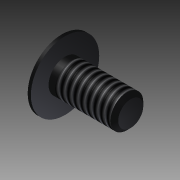
# Autodesk Inventor part: 3342
Saved by Autodesk Inventor 2016 (Build 200138000, 138)
## iProperties
Category: PARTsolutions
Company: 8020
Created: 2016-04-17
Part Number: 3342
Catalog Web Link: www.cadenas.de
Description: 3390, 3342, 3066, 3340, 3330-Flanged Button Head Socket Cap Screws
Vendor: 8020
Document SubType Name: Modeling
Designer: psAdmin
Manufacturer: 8020
Mass: 0.617423 g
Surface Area: 6.01161 cm^2
Volume: 0.617423 cm^3
Density: 1 g/cm^3
Material: Generic
Appearance: PSOLRGB-0-0-0
PSOL_IDENT_0: {$CADENAS_DATA\23d-libs\8020\inch\fastening_options\3390.prj},164 {VTYP=3D},{NB=3342},{LINA=3342},{N
PSOL_IDENT_1: N=3390, 3342, 3066, 3340, 3330},{DATE=22.08.2012},{GEOMDATE=11.05.2012 00:00:00},{VERSION=},{LINEID=
PSOL_IDENT_2: 10},{LINESUBID=-1},{WBVAR=L}  {NB=3342},{LINA=3342},{KT=DUMMY},{PN=3342},{FIN=Black Zinc},{THRD=1/4-
PSOL_IDENT_3: 20},{THRD1=0.2500},{L=0.50000000},{L1=0.375,0.5,0.75},{W=.009},{A=0.120},{D=0.520},{S=0.160},{T=0.09
PSOL_IDENT_4: 0}
NN: 3390, 3342, 3066, 3340, 3330
NT: Flanged Button Head Socket Cap Screws
NB: 3342
NBSYN: $PN.
LINA: 3342
PN: 3342
FIN: Black Zinc
THRD: 1/4-20
L: 1/2
W: .009
SUPPLIER: 8020
ARTICLENO: 3342
BOMINFO: 3342
CREATOR: CADENAS GmbH
Title: 3342
Author: Cadenas PARTsolutions
Comments: Flanged Button Head Socket Cap Screws
Autodesk Inventor part; units mm, degrees
ref_plane "YZ Plane" through (0, 0, 0) normal (1, 0, 0) x (0, 1, 0)
ref_plane "XZ Plane" through (0, 0, 0) normal (0, 1, 0) x (-1, 0, 0)
ref_plane "XY Plane" through (0, 0, 0) normal (0, 0, 1) x (1, 0, 0)
sketch "Sketch_1" plane through (0, 0, 0) normal (0, 0, 1) x (1, 0, 0)
  line L0 (12.7, 0) -> (-3.048, 0)
  line L1 (-3.048, 0) -> (-3.048, 2.4384)
  arc A0 (-0.6096, 5.9436) -> (-3.048, 2.4384) centre (3.3013, 0.6222) ccw
  line L2 (-0.6096, 5.9436) -> (-0.6096, 6.604)
  line L3 (-0.6096, 6.604) -> (0, 6.604)
  line L4 (0, 6.604) -> (0, 3.175)
  line L5 (0, 3.175) -> (11.9444, 3.175)
  line L6 (11.9444, 3.175) -> (12.7, 2.4194)
  line L7 (12.7, 2.4194) -> (12.7, 0)
  line L8 (12.7, 0) -> (-3.048, 0)
  constraints: 18 end point, 2 point on circle, 1 centre point
revolve "Revolution1" add sketch "Sketch_1" angle 360 about axis through (12.7, 0, 0) along (1, 0, 0)
thread "Thread1" size "1/4-20 UNC" class "2A" standard "ANSI Unified Screw Threads" length 10.6355
sketch "Sketch_2" plane through (-3.048, 0, 0) normal (1, 0, 0) x (0, 0, -1)
  line L0 (-2.032, -1.1732) -> (0, -2.3464)
  line L1 (0, -2.3464) -> (2.032, -1.1732)
  line L2 (2.032, -1.1732) -> (2.032, 1.1732)
  line L3 (2.032, 1.1732) -> (0, 2.3464)
  line L4 (0, 2.3464) -> (-2.032, 1.1732)
  line L5 (-2.032, 1.1732) -> (-2.032, -1.1732)
  constraints: 12 end point
extrude "Extrusion1" cut sketch "Sketch_2" along normal blind 2.286
ref_plane "screw_XY" through (0, 0, 0) normal (1, 0, 0) x (0, 0, -1)
ref_plane "screw_YZ" through (0, 0, 0) normal (0, 0, -1) x (0, 1, 0)
ref_plane "screw_ZX" through (0, 0, 0) normal (0, 1, 0) x (1, 0, 0)
ref_plane "to_nut_XY" through (12.7, 0, 0) normal (1, 0, 0) x (0, 0, -1)
ref_plane "to_nut_YZ" through (12.7, 0, 0) normal (0, 0, -1) x (0, 1, 0)
ref_plane "to_nut_ZX" through (12.7, 0, 0) normal (0, 1, 0) x (1, 0, 0)
body "Solid1"
